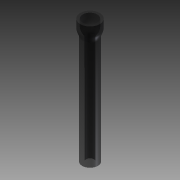
# Autodesk Inventor part: Spring Guide Tube
Saved by Autodesk Inventor 2011 SP2 (Build 150309200, 309)
## iProperties
Created: 2011-07-06
Part Number: Spring Guide Tube
Document SubType Name: Modeling
Designer: sungwook
Density: 1.82 g/cm^3
Material: Viton
Author: sungwook
Autodesk Inventor part; units mm, degrees
ref_plane "YZ Plane" through (0, 0, 0) normal (1, 0, 0) x (0, 1, 0)
ref_plane "XZ Plane" through (0, 0, 0) normal (0, 1, 0) x (-1, 0, 0)
ref_plane "XY Plane" through (0, 0, 0) normal (0, 0, 1) x (1, 0, 0)
sketch "Sketch1" plane through (0, 0, 0) normal (0, 0, 1) x (1, 0, 0)
  circle A0 centre (0, 0) radius 2
  circle A1 centre (0, 0) radius 1
  dimension "d0" = 2
  dimension "d1" = 4
  constraints: 2 centre point, 2 coincident
  measures "d0" diameter of A1
  measures "d1" diameter of A0
extrude "Extrusion1" add sketch "Sketch1" along normal blind 35
sketch "Sketch2" plane through (0, 0, 0) normal (1, 0, 0) x (0, 1, 0)
  line L0 (-2, 35) -> (2, 35) projected
  line L1 (-2, 35) -> (2, 35) projected
  line L2 (-2, 0) -> (2, 0) projected
  line L3 (1, 0) -> (1, 35) projected
  line L4 (2, 0) -> (2, 35) projected
  line L5 (-2, 0) -> (-2, 35) projected
  line L6 (0, -7.8082) -> (0, 46.8491) projected
  line L7 (-1, 0) -> (-1, 35) projected
  spline S0 degree 4 poles (2.5, 37.1511) (2.4385, 36.2785) (2.4715, 36.4932) (2, 35.6037) (2, 35) knots 0 0 0 0 0 1 1 1 1 1
  line L8 (1.85, 39) -> (2.5, 39)
  line L9 (2.5455, 37.7966) -> (2.4545, 36.5056) construction
  arc A0 (2.5379, 37.6674) -> (2.4651, 36.6346) centre (93.2146, 30.7544) ccw construction
  line L10 (1, 35) -> (2, 35)
  spline S1 degree 4 poles (1.85, 39) (1.85, 38.3805) (1.9584, 36.9535) (1.8064, 36.2993) (1, 35.4823) (1, 35) knots 0 0 0 0 0 0.518957 1 1 1 1 1
  line L11 (1.85, 39) -> (1.85, 33.7099)
  spline S2 degree 1 poles (2.5, 39) (2.5, 37.1511) knots 0 0 1 1
  point P0 (0, 0)
  point P1 (2.85, 39)
  point P2 (1.85, 37.1511)
  point P3 (1.4925, 36.0895)
  dimension "d6" = 1
  dimension "d9" = 4
  dimension "d10" = 0.65
  dimension "d11" = 2.5
  constraints: 8 end point, 3 vertical, 2 midpoint, 2 perpendicular, 2 point on line, 1 centre point, 1 collinear, 1 point on circle, 11 other
  measures "d6" distance between parallel lines of L4 L3
  measures "d9" distance between parallel lines of L0 L8
  measures "d10" distance of L8.start L8.end
  measures "d11" distance from line of L8.end L6
revolve "Revolution1" add sketch "Sketch2" angle 360 about axis through (0, 0, -10) along (0, 0, 1) contours S1 L11 L0 | L11 S1 L8 S2 S0 L0
sketch "Sketch3" plane through (0, 0, 0) normal (0, 0, -1) x (-1, 0, 0)
  circle A0 centre (0, 0) radius 2 projected
  circle A1 centre (0, 0) radius 1 projected
  circle A2 centre (0, 0) radius 2
  constraints: 1 centre point, 1 coincident, 1 concentric
extrude "Extrusion2" cut sketch "Sketch3" against normal blind 7.215
equation "\"d0\" = GuideTubingID"
equation "\"d1\" = GuideTubingOD"
equation "\"d10\" = 0.65 * d6"
equation "\"baseOD\" = 23"
equation "\"baseInitD\" = 4"
equation "\"baseTh0\" = 48.463041deg"
equation "\"baseTh1\" = 23.073918deg"
equation "\"topD\" = 14"
equation "\"topInitD\" = 4"
equation "\"topTh0\" = 16.60155deg"
equation "\"topTh1\" = 86.796901deg"
equation "\"dFlexure\" = 0.38"
equation "\"lFlexure\" = 1.5"
equation "\"lFlexureOffset\" = 1.95"
equation "\"dMotor\" = 1.44"
equation "\"lMotor\" = 22.35"
equation "\"topH\" = 21.66629"
equation "\"springBaseD\" = 8"
equation "\"springTopD\" = 8"
equation "\"springInitL\" = 12.7"
equation "\"springLset\" = 3.5"
equation "\"springDeform\" = 18.16629"
equation "\"springL\" = 30.86629"
equation "\"springLO\" = 33.86629"
equation "\"springUnderCut\" = 9.2"
equation "\"dM1X\" = 6.73587"
equation "\"dM1Y\" = 2.34012"
equation "\"dM2X\" = -1.34133"
equation "\"dM2Y\" = 7.00349"
equation "\"dM1Xt\" = 6.59227"
equation "\"dM1Yt\" = -0.43704"
equation "\"dM2Xt\" = -3.67462"
equation "\"dM2Yt\" = 5.49055"
equation "\"GuideRod\" = 2"
equation "\"GuideTubingOD\" = 4"
equation "\"GuideTubingID\" = 2"
equation "\"CSpringOD\" = 5.537"
equation "\"CSpringCD\" = 0.254"
equation "\"CSpringID\" = 5.029"
equation "\"d7\" = d6"
body "Solid1"
